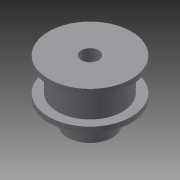
# Autodesk Inventor part: pulley_5mm
Saved by Autodesk Inventor 2015 (Build 190159000, 159)
## iProperties
Created: 2015-08-29
Part Number: pulley_5mm
Material: Generic
Description: insert part description/title
Document SubType Name: Modeling
Designer: francis
Density: 1 g/cm^3
Appearance: Default
Author: francis
Part Category: insert part category here and press enter to fill value
Autodesk Inventor part; units mm, degrees
ref_plane "YZ Plane" through (0, 0, 0) normal (1, 0, 0) x (0, 1, 0)
ref_plane "XZ Plane" through (0, 0, 0) normal (0, 1, 0) x (-1, 0, 0)
ref_plane "XY Plane" through (0, 0, 0) normal (0, 0, 1) x (1, 0, 0)
sketch "Sketch1" plane through (0, 0, 0) normal (1, 0, 0) x (0, 1, 0)
  line L0 (0, 17.5) -> (9.5, 17.5)
  line L1 (9.5, 17.5) -> (9.5, 16)
  line L2 (9.5, 16) -> (6.945, 16)
  line L3 (6.945, 16) -> (6.945, 8)
  line L4 (6.945, 8) -> (9.5, 8)
  line L5 (9.5, 8) -> (9.5, 6.5)
  line L6 (9.5, 6.5) -> (4, 6.5)
  line L7 (4, 6.5) -> (4, 0)
  line L8 (4, 0) -> (0, 0)
  line L9 (0, 0) -> (0, 17.5)
  line L10 (-2.5, 10.0812) -> (-2.5, 1.7277) construction
  dimension "d0" = 24
  dimension "d1" = 17.5
  dimension "d2" = 8
  dimension "d3" = 11
  dimension "d4" = 5
  dimension "d5" = 13
  dimension "d6" = 18.89
  constraints: 22 end point, 8 perpendicular, 2 point on line, 1 collinear, 1 horizontal, 1 vertical
  measures "d0" diameter of L1 L10
  measures "d1" distance between parallel lines of L0 L8
  measures "d2" distance between parallel lines of L4 L2
  measures "d3" distance between parallel lines of L0 L6
  measures "d4" diameter of L9 L10
  measures "d5" diameter of L7 L10
  measures "d6" diameter of L3 L10
revolve "Revolution1" add sketch "Sketch1" angle 360 about axis through (0, -2.5, 10.0812) along (0, 0, -1)
sketch "Sketch2" plane through (0, 0, 0) normal (1, 0, 0) x (0, 1, 0)
  line L0 (-9, 6.5) -> (-9, 0) construction
  line L1 (4, 6.5) -> (4, 0) construction
  line L2 (-9, 0) -> (4, 0) construction
  line L3 (-19.3, 0) -> (14.3, 0) construction
  point P0 (0, 0)
  point P1 (-2.5, 3)
  point P2 (-2.5, 3)
  dimension "d8" = 3
  constraints: 1 coincident
  measures "d8" distance from line of L2 point (-2.5, 3)
hole "Hole1" at (0, -2.5, 3) direction (-1, 0, 0) diameter 2.459 end through all thread size "M3x0.5" class "6H" standard "ISO Metric profile"
body "Solid1"
